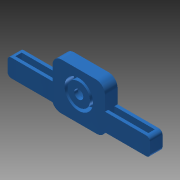
# Autodesk Inventor part: BedClipUltiBotsMiddle
Saved by Autodesk Inventor 2015 SP1 (Build 190203100, 203)
## iProperties
Category: Print
Created: 2013-12-28
Part Number: BedClipUltiBotsMiddle
Material: ABS Plastic
Document SubType Name: Modeling
Designer: Jack
Density: 1.06 g/cm^3
Appearance: Cyan
Mass: 7.19775 g
Surface Area: 54.7331 cm^2
Volume: 6.79033 cm^3
Vendor: Jack
Catalog Web Link: N/A
Author: Jack
Title: Bed Clip Ultibots Center
Autodesk Inventor part; units mm, degrees
ref_plane "YZ Plane" through (0, 0, 0) normal (1, 0, 0) x (0, 1, 0)
ref_plane "XZ Plane" through (0, 0, 0) normal (0, 1, 0) x (-1, 0, 0)
ref_plane "XY Plane" through (0, 0, 0) normal (0, 0, 1) x (1, 0, 0)
sketch "Sketch1" plane through (0, 0, 0) normal (0, 1, 0) x (-1, 0, 0)
  arc A0 (-4.5826, -2) -> (0, -5) centre (0, 0) ccw
  line L0 (47.5826, -2) -> (24.5826, -2)
  arc A1 (20, -5) -> (24.5826, -2) centre (20, 0) ccw
  line L1 (0, -5) -> (20, -5)
  line L2 (49.5826, 0) -> (49.5826, 6)
  line L3 (47.5826, 8) -> (24.5826, 8)
  arc A2 (49.5826, 6) -> (47.5826, 8) centre (47.5826, 6) ccw
  arc A3 (47.5826, -2) -> (49.5826, 0) centre (47.5826, 0) ccw
  line L4 (-4.5826, -2) -> (-27.5826, -2)
  line L5 (-29.5826, 0) -> (-29.5826, 6)
  line L6 (-27.5826, 8) -> (-4.5826, 8)
  line L7 (24.5826, 8) -> (24.5826, 21)
  line L8 (24.5826, 21) -> (-4.5826, 21)
  line L9 (-4.5826, 21) -> (-4.5826, 8)
  arc A4 (-29.5826, 0) -> (-27.5826, -2) centre (-27.5826, 0) ccw
  arc A5 (-27.5826, 8) -> (-29.5826, 6) centre (-27.5826, 6) ccw
  point P0 (49.5826, -2)
  point P1 (49.5826, 8)
  point P2 (-29.5826, -2)
  point P3 (-29.5826, 8)
  dimension "d0" = 5
  dimension "d8" = 5
  dimension "d9" = 20
  dimension "d12" = 3
  dimension "d14" = 10
  dimension "d15" = 2
  dimension "d49" = 25
  dimension "d50" = 25
  dimension "d51" = 10
  dimension "d52" = 26
  dimension "d53" = 2
  constraints: 20 end point, 12 point on circle, 10 tangent, 8 point on line, 6 centre point, 6 perpendicular, 2 equal radius, 2 horizontal alignment, 2 vertical alignment, 1 coincident, 1 horizontal, 1 vertical
  measures "d0" radius of A0
  measures "d8" radius of A1
  measures "d9" distance of point (0, 0) A1.centre
  measures "d12" distance between parallel lines of L1 L0
  measures "d14" distance of point (49.583, -2) point (49.583, 8)
  measures "d15" radius of A2
  measures "d49" distance from line of L0.end L2
  measures "d50" distance of L4.start point (-29.583, -2)
  measures "d51" distance of point (-29.583, -2) point (-29.583, 8)
  measures "d52" vertical distance of L1.start L8.end
  measures "d53" radius of A4
extrude "Extrusion1" add sketch "Sketch1" along normal blind 7
fillet "Fillet2" radius 5 2 edges at (-24.5826, 3.5, 21) (4.5826, 3.5, 21)
sketch "Sketch7" plane through (-24.5826, 0, -2) normal (0, 0, -1) x (-1, 0, 0)
  line L0 (0, 7) -> (23, 7) projected
  line L1 (-52.1652, 0) -> (-29.1652, 0) projected
  line L2 (-29.1652, 0) -> (-29.1652, 7) projected
  line L3 (-52.1652, 7) -> (-29.1652, 7) projected
  line L4 (-52.1652, 0) -> (-52.1652, 7) projected
  line L5 (-51.5652, 1.75) -> (-29.1652, 1.75)
  line L6 (-29.1652, 1.75) -> (-29.1652, 5.25)
  line L7 (-29.1652, 5.25) -> (-51.5652, 5.25)
  line L8 (-51.5652, 5.25) -> (-51.5652, 1.75)
  line L9 (0, 1.75) -> (22.4, 1.75)
  line L10 (22.4, 1.75) -> (22.4, 5.25)
  line L11 (22.4, 5.25) -> (0, 5.25)
  line L12 (0, 5.25) -> (0, 1.75)
  line L13 (-54.1652, 0) -> (-54.1652, 7) projected
  line L14 (25, 0) -> (25, 7) projected
  point P0 (-24.5826, 0)
  dimension "d55" = 22.4
  dimension "d56" = 3.5
  dimension "d57" = 1.75
  dimension "d58" = 2.6
  dimension "d59" = 2.6
  constraints: 16 end point, 4 parallel, 2 equal length, 2 horizontal, 2 perpendicular, 1 horizontal alignment
  measures "d55" distance of L7.end L6.end
  measures "d56" distance of L6.end L5.end
  measures "d57" distance between parallel lines of L0 L11
  measures "d58" distance between parallel lines of L13 L8
  measures "d59" distance between parallel lines of L14 L10
extrude "Extrusion7" cut sketch "Sketch7" against normal up to next contours L5 L8 L7 L2 | L12 L11 L10 L9
sketch "Sketch8" plane through (0, 0, 0) normal (0, -1, 0) x (1, 0, 0)
  line L0 (-24.5826, 8) -> (-24.5826, 16) projected
  line L1 (0, -5) -> (-20, -5) projected
  circle A0 centre (-10.0001, 9) radius 7.925
  circle A1 centre (-10.0001, 9) radius 6.25
  dimension "d62" = 15.85
  dimension "d63" = 14
  dimension "d64" = 12.5
  dimension "d65" = 14.5825
  constraints: 2 centre point, 1 coincident
  measures "d62" diameter of A0
  measures "d63" distance from line of L1 A0.centre
  measures "d64" diameter of A1
  measures "d65" distance from line of L0 A0.centre
extrude "Extrusion8" cut sketch "Sketch8" against normal blind 5
sketch "Sketch9" plane through (-10.0001, 0, 9) normal (0, -1, 0) x (1, 0, 0)
  circle A0 centre (0, 0) radius 6.25 projected
  circle A1 centre (0, 0) radius 2.5
  point P0 (10.0001, -9)
  dimension "d68" = 5
  constraints: 1 centre point, 1 coincident
  measures "d68" diameter of A1
extrude "Extrusion9" cut sketch "Sketch9" against normal up to next contours A1
sketch "Sketch10" plane through (0, 7, 0) normal (0, 1, 0) x (1, 0, 0)
  circle A0 centre (-10.0001, -9) radius 2.5 projected
  circle A1 centre (-10.0001, -9) radius 4.45
  dimension "d71" = 8.9
  constraints: 1 centre point, 1 coincident
  measures "d71" diameter of A1
extrude "Extrusion10" cut sketch "Sketch10" against normal blind 5
sketch "Sketch11" plane through (0, 7, 0) normal (0, 1, 0) x (1, 0, 0)
  arc A0 (4.5826, 2) -> (0, 5) centre (0, 0) ccw projected
  line L0 (0, 5) -> (-20, 5) projected
  arc A1 (-20, 5) -> (-24.5826, 2) centre (-20, 0) ccw projected
  line L1 (-24.5826, 2) -> (-47.5826, 2) projected
  line L2 (4.5826, 2) -> (-24.5826, 2)
  constraints: 2 end point, 1 collinear
extrude "Extrusion11" add sketch "Sketch11" along normal blind 5.5
fillet "Fillet3" radius 1 4 edges at (-22.7386, 12.5, -4.1833) (2.7386, 12.5, -4.1833) (-10, 12.5, -5) (-10, 12.5, -2)
body "Solid1"
